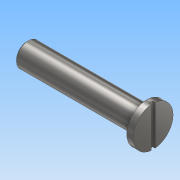
# Autodesk Inventor part: Top_Hinge Cylinder Long
Saved by Autodesk Inventor 2018.1 (Build 221171000, 171)
## iProperties
Created: 2019-03-15
Part Number: Top_Hinge Cylinder Long
Material: Stainless Steel
Document SubType Name: Modeling
Designer: James
Density: 8 g/cm^3
Appearance: Semi-Polished
Author: James
Autodesk Inventor part; units mm, degrees
ref_plane "YZ Plane" through (0, 0, 0) normal (1, 0, 0) x (0, 1, 0)
ref_plane "XZ Plane" through (0, 0, 0) normal (0, 1, 0) x (-1, 0, 0)
ref_plane "XY Plane" through (0, 0, 0) normal (0, 0, 1) x (1, 0, 0)
sketch "Sketch1" plane through (0, 0, 0) normal (0, 0, 1) x (1, 0, 0)
  line L0 (0, 0) -> (150, 0)
  line L1 (150, 0) -> (150, 15)
  line L2 (150, 15) -> (0, 15)
  line L3 (0, 15) -> (0, 0)
  line L4 (150, 0) -> (158, 0)
  line L5 (158, 0) -> (158, 25)
  line L6 (158, 25) -> (150, 25)
  line L7 (150, 25) -> (150, 0)
  dimension "d0" = 15
  dimension "d1" = 25
  dimension "d2" = 150
  dimension "d3" = 8
  constraints: 16 end point, 4 parallel, 2 horizontal, 2 perpendicular
  measures "d0" distance of L2.end L0.start
  measures "d1" distance of L4.end L5.end
  measures "d2" distance of L1.end L2.end
  measures "d3" distance of L5.end L6.end
revolve "Revolution1" add sketch "Sketch1" angle 360 about axis through (0, 0, 0) along (1, 0, 0)
fillet "Fillet1" radius 3 1 edges at (150, -15, 0)
chamfer "Chamfer1" distance 2 angle 45 1 edges at (0, -15, 0)
sketch "Sketch2" plane through (0, 0, 0) normal (-1, 0, 0) x (0, 0, 1)
  point P0 (0, 0)
  point P1 (0, 0)
  constraints: 1 coincident
hole "Hole1" at (0, 0, 0) direction (1, 0, 0) diameter 6.647 depth 22.2 tip angle 118 thread size "M8x1.25" class "6H" standard "ANSI Metric M Profile"
sketch "Sketch3" plane through (158, 0, 0) normal (1, 0, 0) x (0, 0, -1)
  line L0 (-25, 2.5) -> (25, 2.5)
  line L1 (25, 2.5) -> (25, -2.5)
  line L2 (25, -2.5) -> (-25, -2.5)
  line L3 (-25, -2.5) -> (-25, 2.5)
  circle A0 centre (0, 0) radius 18 projected
  circle A1 centre (0, 0) radius 25 projected
  dimension "d16" = 50
  dimension "d17" = 50
  dimension "d18" = 25
  dimension "d19" = 5
  dimension "d20" = 2.5
  constraints: 8 end point, 2 parallel, 1 horizontal, 1 perpendicular
  measures "d16" diameter of A1
  measures "d17" distance of L0.start L0.end
  measures "d18" distance from line of L1 point (0, 0)
  measures "d19" distance of L0.end L1.end
  measures "d20" distance from line of point (0, 0) L0
extrude "Extrusion1" cut sketch "Sketch3" against normal blind 3 contours L0 A1 L3 | L0 A0 L2 A1 | A1 L2 L3 | L0 A0 L2 | A1 L2 A0 L0 | L0 L1 A1 | L1 L2 A1
equation "\"d17\" = d16"
equation "\"d18\" = 0.5 * d17"
equation "\"d20\" = 0.5 * d19"
body "Solid1"
